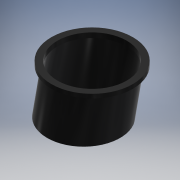
# Autodesk Inventor part: Water Bottle Ring
Saved by Autodesk Inventor 2019 (Build 230136000, 136)
## iProperties
Created: 2020-12-25
Part Number: Water Bottle Ring
Material: Acetal Resin, Black
Document SubType Name: Modeling
Designer: John
Density: 1.425 g/cm^3
Appearance: Smooth - Black
Author: John
Autodesk Inventor part; units mm, degrees
ref_plane "YZ Plane" through (0, 0, 0) normal (1, 0, 0) x (0, 1, 0)
ref_plane "XZ Plane" through (0, 0, 0) normal (0, 1, 0) x (-1, 0, 0)
sketch "Sketch1" plane through (0, 0, 0) normal (0, 1, 0) x (-1, 0, 0)
  circle A0 centre (0, 0) radius 63.5
  circle A1 centre (0, 0) radius 57.15
  circle A2 centre (0, 0) radius 50.8 construction
  circle A3 centre (0, 0) radius 53.975
  dimension "d1" = 127
  dimension "d2" = 114.3
  dimension "d3" = 101.6
  dimension "d4" = 107.95
  constraints: 4 centre point, 3 coincident
  measures "d1" diameter of A0
  measures "d2" diameter of A1
  measures "d3" diameter of A2
  measures "d4" diameter of A3
extrude "Extrusion1" add sketch "Sketch1" along normal blind 6.35 contours A0 | A1
extrude "Extrusion2" add sketch "Sketch1" against normal blind 25.4 contours A1
sketch "Sketch2" plane through (0, 0, 0) normal (0, 0, 1) x (1, 0, 0)
  line L0 (-57.15, -25.4) -> (57.15, -25.4) projected
  line L1 (-57.15, -25.4) -> (-57.15, -50.8)
  line L2 (-57.15, -25.4) -> (-31.75, -25.4) construction
  point P0 (0, 0)
  dimension "d9" = 90
  dimension "d10" = 25.4
  constraints: 4 end point, 1 horizontal, 1 perpendicular
  measures "d9" angle of L1 L2
  measures "d10" distance of L0.start L1.end
ref_plane "Work Plane1" through (-57.15, -50.8, 0) normal (0, -1, 0) x (1, 0, 0)
body "Solid1"
